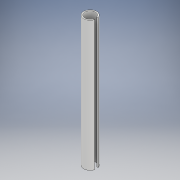
# Autodesk Inventor part: outer_sheath
Saved by Autodesk Inventor 2017 (Build 210142000, 142)
## iProperties
Created: 2018-11-30
Part Number: outer_sheath
Material: Acetal Resin, White
Document SubType Name: Modeling
Designer: ddeboer
Density: 1.425 g/cm^3
Appearance: Smooth - White
Author: ddeboer
Autodesk Inventor part; units mm, degrees
ref_plane "YZ Plane" through (0, 0, 0) normal (1, 0, 0) x (0, 1, 0)
ref_plane "XZ Plane" through (0, 0, 0) normal (0, 1, 0) x (-1, 0, 0)
ref_plane "XY Plane" through (0, 0, 0) normal (0, 0, 1) x (1, 0, 0)
sketch "Sketch1" plane through (0, 0, 0) normal (0, 0, 1) x (1, 0, 0)
  circle A0 centre (0, 0) radius 21.08
  circle A1 centre (0, 0) radius 17.35
  dimension "d0" = 42.16
  dimension "d1" = 3.73
  constraints: 2 centre point, 1 coincident
  measures "d0" diameter of A0
  measures "d1" radial gap between concentric circles of A1 A0
extrude "Extrusion1" add sketch "Sketch1" along normal blind 425
sketch "Sketch2" plane through (0, 0, 425) normal (0, 0, 1) x (1, 0, 0)
  line L0 (20.2483, -11.9795) -> (24.1852, -11.9795)
  line L1 (24.1852, -11.9795) -> (24.1852, 11.4148)
  line L2 (24.1852, 11.4148) -> (20.2483, 11.4148)
  line L3 (20.2483, 11.4148) -> (20.2483, -11.9795)
  point P0 (0, 0)
  constraints: 8 end point, 2 parallel, 1 horizontal, 1 perpendicular
extrude "Extrusion2" cut sketch "Sketch2" against normal blind 500
sketch "Sketch4" plane through (20.2483, -5.8629, 425) normal (1, 0, 0) x (0, 0, -1)
  line L0 (425, 23.2129) -> (425, -11.4871) projected
  line L1 (0, 11.7258) -> (425, 11.7258) projected
  line L2 (425, 0.0315) -> (0, 0.0315)
  line L3 (0, 0.0315) -> (0, 11.7258)
  line L4 (0, 11.7258) -> (425, 11.7258)
  line L5 (425, 11.7258) -> (425, 0.0315)
  point P0 (425, 5.8629)
  constraints: 8 end point, 2 parallel, 1 horizontal, 1 perpendicular, 1 point on line
extrude "Extrusion3" cut sketch "Sketch4" against normal blind 10
body "Solid1"
